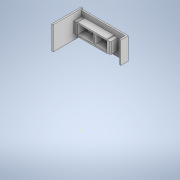
# Autodesk Inventor part: basecaixa
Saved by Autodesk Inventor 2022 (Build 260153000, 153)
## iProperties
Created: 2024-03-03
Part Number: basecaixa
Material: Genérico
Document SubType Name: Modeling
Designer: Daniel
Density: 1 g/cm^3
Appearance: Padrão
Author: Daniel
Autodesk Inventor part; units mm, degrees
ref_plane "YZ Plane" through (0, 0, 0) normal (1, 0, 0) x (0, 1, 0)
ref_plane "XZ Plane" through (0, 0, 0) normal (0, 1, 0) x (-1, 0, 0)
ref_plane "XY Plane" through (0, 0, 0) normal (0, 0, 1) x (1, 0, 0)
sketch "Esboço1" plane through (0, 0, 0) normal (0, 0, 1) x (1, 0, 0)
  line L0 (0, 0) -> (60, 0)
  line L1 (60, 0) -> (60, 110)
  line L2 (60, 110) -> (0, 110)
  line L3 (0, 110) -> (0, 0)
  line L4 (62, 112) -> (62, -2)
  line L5 (62, -2) -> (-2, -2)
  line L6 (-2, -2) -> (-2, 112)
  line L7 (-2, 112) -> (62, 112)
  dimension "d0" = 60
  dimension "d1" = 110
  dimension "d2" = 2
  constraints: 16 end point, 4 parallel, 2 perpendicular, 1 horizontal, 3 other
  measures "d0" distance of L2.end L1.end
  measures "d1" distance of L0.end L1.end
  measures "d2" distance between parallel lines of L1 L4
extrude "Extrusão1" add sketch "Esboço1" along normal blind 2 contours L3 L2 L1 L0 | L4 L5 L6 L7
sketch "Esboço2" plane through (0, 0, 2) normal (0, 0, 1) x (1, 0, 0)
  line L0 (62, 112) -> (-2, 112) projected
  line L1 (-2, 112) -> (-2, -2) projected
  line L2 (62, -2) -> (62, 112) projected
  line L3 (-2, -2) -> (62, -2) projected
  line L4 (0, 0) -> (0, 110)
  line L5 (0, 110) -> (60, 110)
  line L6 (60, 110) -> (60, 0)
  line L7 (60, 0) -> (0, 0)
  point P0 (0, 0)
  dimension "d5" = 2
  constraints: 8 end point, 3 other
  measures "d5" distance between parallel lines of L1 L4
extrude "Extrusão2" add sketch "Esboço2" along normal blind 38
sketch "Esboço3" plane through (-2, -2, 0) normal (0, -1, 0) x (1, 0, 0)
  line L0 (32, 5) -> (42, 5)
  line L1 (42, 5) -> (42, 15)
  line L2 (42, 15) -> (32, 15)
  line L3 (32, 15) -> (32, 5)
  line L4 (0, 0) -> (64, 0) projected
  line L5 (64, 0) -> (64, 40) projected
  point P0 (2, 0)
  dimension "d8" = 10
  dimension "d9" = 10
  dimension "d10" = 5
  dimension "d11" = 22
  constraints: 8 end point, 2 parallel, 1 horizontal, 1 perpendicular
  measures "d8" distance of L0.end L1.end
  measures "d9" distance of L1.end L2.end
  measures "d10" distance between parallel lines of L4 L0
  measures "d11" distance between parallel lines of L5 L1
extrude "Extrusão3" cut sketch "Esboço3" against normal blind 38
sketch "Esboço11" plane through (-2, 112, 0) normal (0, 1, 0) x (1, 0, 0)
  line L0 (64, 0) -> (64, -40) projected
  line L1 (0, 0) -> (64, 0)
  line L2 (64, 0) -> (64, -2)
  line L3 (64, -2) -> (0, -2)
  line L4 (0, -2) -> (0, 0)
  line L5 (64, 0) -> (0, 0) projected
  point P0 (2, 0)
  dimension "d45" = 2
  dimension "d46" = 0
  dimension "d47" = 64
  constraints: 8 end point, 2 parallel, 1 horizontal, 1 perpendicular, 1 point on line
  measures "d45" distance of L3.end L1.start
  measures "d46" distance between parallel lines of L5 L1
  measures "d47" distance between parallel lines of L4 L0
extrude "Extrusão8" add sketch "Esboço11" along normal blind 32
sketch "Esboço12" plane through (-2, 112, 2) normal (0, 0, 1) x (1, 0, 0)
  line L0 (2, 7.5) -> (7, 7.5)
  line L1 (7, 7.5) -> (7, 22.5)
  line L2 (7, 22.5) -> (2, 22.5)
  line L3 (2, 22.5) -> (2, 7.5)
  line L4 (52, 7.5) -> (47, 7.5)
  line L5 (47, 7.5) -> (47, 22.5)
  line L6 (47, 22.5) -> (52, 22.5)
  line L7 (52, 22.5) -> (52, 7.5)
  line L8 (64, 0) -> (0, 0) projected
  line L9 (0, 0) -> (0, 32) projected
  point P0 (2, -112)
  dimension "d50" = 5
  dimension "d51" = 15
  dimension "d52" = 5
  dimension "d53" = 15
  dimension "d54" = 7.5
  dimension "d55" = 7.5
  dimension "d56" = 40
  dimension "d57" = 2
  constraints: 16 end point, 4 parallel, 2 horizontal, 2 perpendicular
  measures "d50" distance of L2.end L1.end
  measures "d51" distance of L1.end L0.end
  measures "d52" distance of L5.end L6.end
  measures "d53" distance of L4.end L5.end
  measures "d54" distance between parallel lines of L8 L0
  measures "d55" distance between parallel lines of L8 L4
  measures "d56" distance between parallel lines of L1 L5
  measures "d57" distance between parallel lines of L9 L3
extrude "Extrusão9" add sketch "Esboço12" along normal blind 10
sketch "Esboço13" plane through (-2, 112, 2) normal (0, 0, 1) x (1, 0, 0)
  circle A0 centre (17, 15) radius 1.5
  circle A1 centre (17, 15) radius 2
  circle A2 centre (17, 15) radius 3.5
  line L0 (7, 7.5) -> (7, 22.5) projected
  line L1 (0, 32) -> (64, 32) projected
  point P0 (2, -112)
  dimension "d60" = 3
  dimension "d61" = 4
  dimension "d62" = 7
  dimension "d69" = 10
  dimension "d70" = 17
  constraints: 3 centre point, 2 coincident
  measures "d60" diameter of A0
  measures "d61" diameter of A1
  measures "d62" diameter of A2
  measures "d69" distance from line of L0 A2.centre
  measures "d70" distance from line of L1 A2.centre
extrude "Extrusão10" add sketch "Esboço13" along normal blind 3 contours A2
fillet "Arredondamento1" radius 3.5 1 edges at (13, 127, 5)
sketch "Esboço14" plane through (15, 127, 2) normal (0, 0, 1) x (1, 0, 0)
  circle A0 centre (0, 0) radius 1.5
  point P0 (-15, -127)
  dimension "d66" = 3
  constraints: 1 centre point
  measures "d66" diameter of A0
extrude "Extrusão11" cut sketch "Esboço14" against normal blind 3
sketch "Esboço16" plane through (-2, 112, 2) normal (0, 0, 1) x (1, 0, 0)
  line L0 (47, 22.5) -> (47, 7.5) projected
  line L1 (7, 6.5) -> (47, 6.5)
  line L2 (47, 6.5) -> (47, 8.5)
  line L3 (47, 8.5) -> (7, 8.5)
  line L4 (7, 8.5) -> (7, 6.5)
  line L5 (7, 7.5) -> (7, 22.5) projected
  line L6 (47, 23.5) -> (7, 23.5)
  line L7 (7, 23.5) -> (7, 21.5)
  line L8 (7, 21.5) -> (47, 21.5)
  line L9 (47, 21.5) -> (47, 23.5)
  circle A0 centre (17, 15) radius 1.5 projected
  point P0 (2, -112)
  point P1 (47, 21.5)
  dimension "d77" = 2
  dimension "d78" = 2
  dimension "d79" = 13
  dimension "d80" = 6.5
  dimension "d81" = 40
  constraints: 16 end point, 4 parallel, 3 point on line, 2 horizontal, 2 perpendicular
  measures "d77" distance of L3.end L1.start
  measures "d78" distance of L6.end L7.end
  measures "d79" distance between parallel lines of L3 L8
  measures "d80" distance from line of L3 A0.centre
  measures "d81" distance of L1.start L1.end
extrude "Extrusão13" add sketch "Esboço16" along normal blind 10 contours L0 L8 L5 L7 L6 L9 | L0 L2 L1 L4 L3
sketch "Esboço17" plane through (5, 133.5, 2) normal (0, 0, 1) x (1, 0, 0)
  line L0 (0, 0) -> (40, 0) projected
  line L1 (23.5, 0) -> (21.5, 0)
  line L2 (21.5, 0) -> (21.5, -13)
  line L3 (21.5, -13) -> (23.5, -13)
  line L4 (23.5, -13) -> (23.5, 0)
  line L5 (40, -13) -> (0, -13) projected
  circle A0 centre (10, -6.5) radius 1.5 projected
  point P0 (-5, -133.5)
  point P1 (21.5, 0)
  dimension "d84" = 0
  dimension "d85" = 2
  dimension "d86" = 10
  constraints: 8 end point, 2 parallel, 1 horizontal, 1 perpendicular, 1 point on line
  measures "d84" distance between parallel lines of L5 L3
  measures "d85" distance between parallel lines of L4 L2
  measures "d86" distance edge to line of A0 L2
extrude "Extrusão14" add sketch "Esboço17" along normal blind 10 contours L0 L4 L3 L2
sketch "Esboço18" plane through (-2, 112, 2) normal (0, 0, 1) x (1, 0, 0)
  line L0 (30.5, 21.5) -> (30.5, 8.5) projected
  line L1 (30.5, 8.5) -> (47, 8.5) projected
  line L2 (47, 8.5) -> (47, 21.5) projected
  line L3 (47, 21.5) -> (30.5, 21.5) projected
  line L4 (28.5, 8.5) -> (28.5, 21.5) projected
  line L5 (28.5, 21.5) -> (7, 21.5) projected
  line L6 (7, 21.5) -> (7, 8.5) projected
  line L7 (7, 8.5) -> (28.5, 8.5) projected
  circle A0 centre (17, 15) radius 1.5 projected
  circle A1 centre (17, 15) radius 2 projected
  circle A2 centre (17, 15) radius 3.5 projected
  line L8 (52, 22.5) -> (52, 7.5) projected
  line L9 (52, 7.5) -> (47, 7.5) projected
  line L10 (47, 7.5) -> (47, 6.5) projected
  line L11 (47, 6.5) -> (7, 6.5) projected
  line L12 (7, 6.5) -> (7, 7.5) projected
  line L13 (7, 7.5) -> (2, 7.5) projected
  line L14 (2, 7.5) -> (2, 22.5) projected
  line L15 (2, 22.5) -> (7, 22.5) projected
  line L16 (7, 22.5) -> (7, 23.5) projected
  line L17 (7, 23.5) -> (47, 23.5) projected
  line L18 (47, 23.5) -> (47, 22.5) projected
  line L19 (47, 22.5) -> (52, 22.5) projected
  line L20 (0, 0) -> (64, 0) projected
  line L21 (64, 32) -> (64, 0) projected
  line L22 (0, 32) -> (64, 32) projected
  line L23 (0, 0) -> (0, 32) projected
  line L24 (0, -114) -> (0, 0) projected
  line L25 (64, -114) -> (0, -114) projected
  line L26 (64, 0) -> (64, -114) projected
  line L27 (2, -112) -> (62, -112) projected
  line L28 (62, -112) -> (62, -2) projected
  line L29 (62, -2) -> (2, -2) projected
  line L30 (2, -2) -> (2, -112) projected
  line L31 (62, 0) -> (62, 30)
  line L32 (62, 30) -> (2, 30)
  line L33 (2, 30) -> (2, 0)
  point P0 (2, 7.5)
  dimension "d89" = 2
  constraints: 6 end point, 2 other
  measures "d89" distance between parallel lines of L22 L32
extrude "Extrusão15" add sketch "Esboço18" along normal blind 38 contours L14 L33 L20 L23 L22 L21 L31 L32
sketch "Esboço19" plane through (62, -2, 40) normal (1, 0, 0) x (0, 0, -1)
  line L0 (30, 144) -> (0, 144)
  line L1 (0, 144) -> (0, 114)
  line L2 (0, 114) -> (30, 114)
  line L3 (30, 114) -> (30, 144)
  line L4 (40, 0) -> (40, 146) projected
  line L5 (40, 146) -> (0, 146) projected
  line L6 (0, 0) -> (0, 146) projected
  point P0 (40, 2)
  dimension "d92" = 10
  dimension "d93" = 2
  dimension "d94" = 0
  dimension "d95" = 30
  constraints: 8 end point, 2 parallel, 1 horizontal, 1 perpendicular
  measures "d92" distance between parallel lines of L4 L3
  measures "d93" distance between parallel lines of L5 L0
  measures "d94" distance between parallel lines of L6 L1
  measures "d95" distance of L2.end L0.start
extrude "Extrusão16" cut sketch "Esboço19" against normal blind 2
chamfer "Chanfro1" distance 1.5 angle 45 1 edges at (50, 127, 12)
sketch "Esboço20" plane through (-2, -2, 0) normal (-1, 0, 0) x (0, 0, 1)
  line L0 (25, 86) -> (15, 86)
  line L1 (15, 86) -> (15, 96)
  line L2 (15, 96) -> (25, 96)
  line L3 (25, 96) -> (25, 86)
  line L4 (0, 146) -> (40, 146) projected
  line L5 (0, 146) -> (0, 0) projected
  point P0 (0, 2)
  dimension "d101" = 10
  dimension "d102" = 10
  dimension "d103" = 50
  dimension "d104" = 15
  constraints: 8 end point, 2 parallel, 1 horizontal, 1 perpendicular
  measures "d101" distance of L0.end L1.end
  measures "d102" distance of L1.end L2.end
  measures "d103" distance between parallel lines of L4 L2
  measures "d104" distance between parallel lines of L5 L1
extrude "Extrusão17" cut sketch "Esboço20" against normal blind 2
sketch "Esboço21" plane through (0, 0, 2) normal (0, 0, 1) x (1, 0, 0)
  point P0 (0, 0)
sketch "Esboço22" plane through (0, 0, 2) normal (0, 0, 1) x (1, 0, 0)
  line L0 (110.309, -33.0792) -> (-25.5735, -33.0792)
  line L1 (-25.5735, -33.0792) -> (-25.5735, 112)
  line L2 (-25.5735, 112) -> (110.309, 112)
  line L3 (110.309, 112) -> (110.309, -33.0792)
  line L4 (62, 112) -> (0, 112) projected
  point P0 (0, 0)
  dimension "d107" = 0
  constraints: 8 end point, 2 parallel, 1 horizontal, 1 perpendicular
  measures "d107" distance between parallel lines of L4 L2
extrude "Extrusão18" cut sketch "Esboço22" along normal mid plane 100
sketch "Esboço23" plane through (50, 119.5, 2) normal (0, 0, 1) x (1, 0, 0)
  line L0 (12, 24.5) -> (-52, 24.5) projected
  line L1 (12, 22.5) -> (-50, 22.5)
  line L2 (-50, 22.5) -> (-50, 24.5)
  line L3 (-50, 24.5) -> (12, 24.5)
  line L4 (12, 24.5) -> (12, 22.5)
  point P0 (-50, -119.5)
  constraints: 8 end point, 2 parallel, 1 horizontal, 1 perpendicular, 1 point on line
extrude "Extrusão19" cut sketch "Esboço23" along normal mid plane 100
